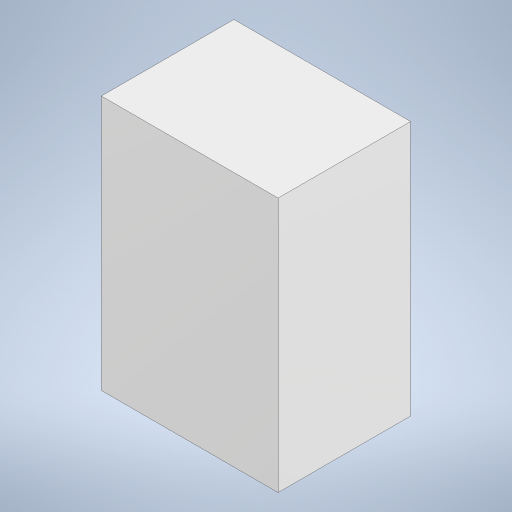
# Autodesk Inventor part: Dishwasher
Saved by Autodesk Inventor 2024 (Build 280153000, 153)
## iProperties
Created: 2023-03-29
Part Number: Dishwasher
Material: ABS Plastic
Document SubType Name: Modeling
Designer: Tom
Density: 1.06 g/cm^3
Appearance: Smooth - White
Author: Tom
Autodesk Inventor part; units mm, degrees
ref_plane "YZ Plane" through (0, 0, 0) normal (1, 0, 0) x (0, 1, 0)
ref_plane "XZ Plane" through (0, 0, 0) normal (0, 1, 0) x (-1, 0, 0)
ref_plane "XY Plane" through (0, 0, 0) normal (0, 0, 1) x (1, 0, 0)
sketch "Sketch1" plane through (0, 0, 0) normal (0, 1, 0) x (-1, 0, 0)
  line L0 (0, 0) -> (-609.6, 0)
  line L1 (-609.6, 0) -> (-609.6, -457.2)
  line L2 (-609.6, -457.2) -> (0, -457.2)
  line L3 (0, -457.2) -> (0, 0)
  dimension "d6" = 457.2
  dimension "d8" = 609.6
  constraints: 8 end point, 2 parallel, 1 horizontal, 1 perpendicular
  measures "d6" distance of L2.end L0.start
  measures "d8" distance of L1.end L2.end
extrude "Extrusion1" add sketch "Sketch1" along normal blind 879.475
body "Solid1"
